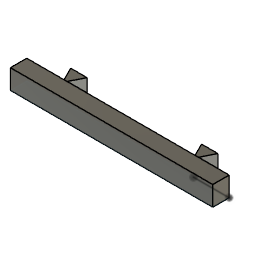
Simply supported beam (Autodesk Fusion 360 design; units mm, degrees)
Autodesk Fusion 360 part; units mm, degrees
sketch "Sketch1" plane through (0, 0, 0) normal (0, 1, 0) x (1, 0, 0)
  line L0 (0, 0) -> (368.8231, 0)
  line L1 (368.8231, 0) -> (368.8231, -35.9552)
  line L2 (368.8231, -35.9552) -> (0, -35.9552)
  line L3 (0, -35.9552) -> (0, 0)
  constraint horizontal L0
  constraint vertical L1
  constraint horizontal L2
  constraint vertical L3
  constraint coincident L0.start L3.end
extrude "Extrude1" add sketch "Sketch1" against normal blind 30 makes body 1
sketch "Sketch2" plane through (0, 0, 0) normal (0, 0, -1) x (1, 0, 0)
  line L0 (0, 0) -> (368.8231, 0)
  line L1 (368.8231, 0) -> (368.8231, 30)
  line L2 (368.8231, 30) -> (0, 30)
  line L3 (0, 30) -> (0, 0)
  line L4 (50, -30) -> (65, 0)
  line L5 (65, 0) -> (80, -30)
  line L6 (80, -30) -> (50, -30)
  constraint coincident L0 L4.end
  constraint parallel L0 L6
extrude "Extrude2" add sketch "Sketch2" along normal blind -26 and the other way blind 0 separate body contours L4 L5 L6 makes body 2
move_body "Move1" bodies 2 to x (1, 0, 0) y (0, 1, 0) z (0, 0, 1) at (0, 0, 4.2595)
sketch "Sketch3" plane through (0, 0, 0) normal (0, 0, -1) x (1, 0, 0)
  line L0 (0, 0) -> (368.8231, 0)
  line L1 (368.8231, 0) -> (368.8231, 30)
  line L2 (368.8231, 30) -> (0, 30)
  line L3 (0, 30) -> (0, 0)
  line L4 (368.8231, 0) -> (303.8231, 0)
  dimension "d7" = 65
  constraint coincident L0.end L1.start
  constraint coincident L0 L4.end
  measures "d7" distance of L0.end L4.end
copy_body "CopyPasteBodies1" bodies 2 makes body 3
move_body "Move2" bodies 3 to x (1, 0, 0) y (0, 1, 0) z (0, 0, 1) at (238.9583, -0.5512, 0)
